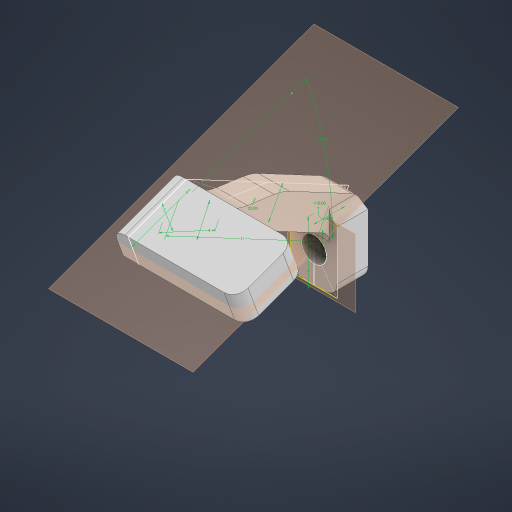
# Autodesk Inventor part: battery-stopper-1
Saved by Autodesk Inventor 2023.5 (Build 275446000, 446)
## iProperties
Created: 2025-02-09
Part Number: battery-stopper-1
Material: 一般
Document SubType Name: Modeling
Designer: IshiiLabHonda
Density: 1 g/cm^3
Appearance: 既定
Author: IshiiLabHonda
Autodesk Inventor part; units mm, degrees
ref_plane "YZ Plane" through (0, 0, 0) normal (1, 0, 0) x (0, 1, 0)
ref_plane "XZ Plane" through (0, 0, 0) normal (0, 1, 0) x (-1, 0, 0)
ref_plane "XY Plane" through (0, 0, 0) normal (0, 0, 1) x (1, 0, 0)
sketch "スケッチ5" plane through (0, 0, 0) normal (1, 0, 0) x (0, 1, 0)
  line L0 (0, 0) -> (0, 1.2936) construction
  line L1 (0, 0) -> (-1.3338, 0) construction
  line L2 (2, 2) -> (-2, 2)
  line L3 (-2, 2) -> (-2, 0)
  line L4 (-2, 0) -> (2, 0)
  line L5 (2, 0) -> (2, 2)
  line L6 (0.8, 2) -> (0.8, 0)
  line L7 (-0.8, 2) -> (-0.8, 0)
  line L8 (-2, 1) -> (2, 1) construction
  line L9 (2, 1) -> (7.1642, 10.7124) construction
  line L10 (8.0471, 10.243) -> (6.2812, 11.1819)
  line L11 (6.2812, 11.1819) -> (0.7025, 0.6899)
  line L12 (0.7025, 0.6899) -> (2.4684, -0.2491)
  line L13 (2.4684, -0.2491) -> (8.0471, 10.243)
  line L14 (2, 0) -> (2.6009, 0)
  line L15 (6.6791, 14.0017) -> (4.7997, 13.3177)
  line L16 (4.7997, 13.3177) -> (6.1677, 9.5589)
  line L17 (6.1677, 9.5589) -> (8.0471, 10.243)
  line L18 (8.0471, 10.243) -> (6.6791, 14.0017)
  line L19 (6.6791, 14.0017) -> (6.1677, 9.5589) construction
  line L20 (4.7997, 13.3177) -> (8.0471, 10.243) construction
  line L21 (5.7394, 13.6597) -> (7.1074, 9.9009) construction
  line L22 (6.4234, 11.7803) -> (4.7515, 8.1465) construction
  line L23 (4.7515, 8.1465) -> (4.3748, 5.4664) construction
  line L24 (6.2812, 11.1819) -> (2.4684, -0.2491) construction
  line L25 (0.7025, 0.6899) -> (8.0471, 10.243) construction
  line L26 (7.3319, 11.3623) -> (5.5149, 12.1983)
  line L27 (5.5149, 12.1983) -> (3.843, 8.5645)
  line L28 (3.843, 8.5645) -> (5.66, 7.7285)
  line L29 (5.66, 7.7285) -> (7.3319, 11.3623)
  line L30 (7.3319, 11.3623) -> (3.843, 8.5645) construction
  line L31 (5.5149, 12.1983) -> (5.66, 7.7285) construction
  line L32 (5.66, 7.7285) -> (5.2826, 5.0437)
  line L33 (3.843, 8.5645) -> (2.6532, 0.0985)
  line L34 (3.467, 5.8892) -> (5.2329, 4.9502)
  point P0 (1.3991, 2)
  point P1 (5.5874, 9.9634)
  point P2 (5.3431, 11.8247)
  point P3 (6.5694, 9.7051)
  dimension "d25" = 1.6
  dimension "d26" = 4
  dimension "d27" = 2
  dimension "d28" = 118
  dimension "d29" = 2
  dimension "d30" = 11
  dimension "d44" = 2
  dimension "d45" = 20
  dimension "d46" = 4
  dimension "d52" = 20
  dimension "d53" = 4
  dimension "d54" = 2
  constraints: 70 end point, 15 midpoint, 15 point on line, 10 parallel, 7 perpendicular, 1 coincident, 1 vertical, 6 other
  measures "d25" distance between parallel lines of L7 L6
  measures "d26" distance between parallel lines of L3 L5
  measures "d27" distance between parallel lines of L4 L2
  measures "d28" angle of L8 L9
  measures "d29" distance between parallel lines of L13 L11
  measures "d30" distance of L8.end L9.end
  measures "d44" distance between parallel lines of L18 L16
  measures "d45" angle of L0 L21
  measures "d46" distance between parallel lines of L17 L15
  measures "d52" angle of L9 L23
  measures "d53" distance of L22.start L22.end
  measures "d54" distance between parallel lines of L29 L27
extrude "押し出し8" add sketch "スケッチ5" along normal mid plane 3 contours L6 L11 L12 L4 L7 L2 | L2 L11 L6 | L7 L4 L3 L2 | L2 L5 L12 L6 L11 | L6 L12 L11 | L12 L4 L6
ref_plane "作業平面7" through (-1.5, -2, 2) normal (0, 0, 1) x (1, 0, 0)
sketch "スケッチ6" plane through (-1.5, -2, 2) normal (0, 0, 1) x (1, 0, 0)
  line L0 (3, 0) -> (0, 0) projected
  line L1 (3, 4) -> (3, 0) projected
  line L2 (0, 4) -> (3, 4) projected
  line L3 (0, 0) -> (0, 4) projected
  line L4 (0, 4) -> (3, 4) projected
  line L5 (0, 4) -> (3, 0) construction
  line L6 (0, 0) -> (3, 0) projected
  line L7 (3, 0) -> (3, 4) projected
  line L8 (0, 0) -> (3, 4) construction
  circle A0 centre (1.5, 2) radius 0.8
  dimension "d35" = 1.6
  constraints: 4 end point, 1 centre point, 1 coincident
  measures "d35" diameter of A0
extrude "押し出し9" cut sketch "スケッチ6" against normal blind 4 contours A0
extrude "押し出し13" add sketch "スケッチ5" along normal blind 7 contours L16 L27 L26 L29 L10 L11 | L11 L10 L29 L17 L16 | L16 L15 L18 L10 L29 L26 L27 | L29 L10 L17
extrude "押し出し15" add sketch "スケッチ5" along normal mid plane 2 contours L11 L33 L13 L14 L5 L2 | L33 L28 L11 | L34 L13 L33 | L11 L28 L32 L13 L34 | L28 L27 L16 L11 | L11 L16 L17 L29 L28 | L16 L27 L26 L29 L10 L11 | L11 L10 L29 L17 L16
extrude "押し出し16" add sketch "スケッチ5" against normal blind 1 contours L16 L15 L18 L10 L29 L26 L27 | L29 L10 L17
fillet "フィレット1" radius 0.8 1 edges at (0, 1.3991, 2)
fillet "フィレット2" radius 1 1 edges at (0, 2.6009, 0)
fillet "フィレット3" radius 3 4 edges at (0, 5.2826, 5.0437) (0, 3.467, 5.8892) (0, 3.843, 8.5645) (0, 5.66, 7.7285)
fillet "フィレット4" radius 3 2 edges at (0, 5.3431, 11.8247) (0, 6.5694, 9.7051)
fillet "フィレット6" radius 0.8 1 edges at (-1, 7.3631, 12.1223)
ref_plane "作業平面8" through (-0.2, 5.7394, 13.6597) normal (0, 0.9396926, 0.3420201) x (1, 0, 0)
sketch "スケッチ8" plane through (-0.2, 5.7394, 13.6597) normal (0, 0.9396926, 0.3420201) x (1, 0, 0)
  point P0 (0.2, 10.8729)
fillet "フィレット11" radius 0.8 2 edges at (7, 5.7394, 13.6597) (7, 7.1074, 9.9009)
fillet "フィレット12" radius 0.8 4 edges at (1, 2, 1) (-1, 2, 1) (-1.5, -2, 1) (1.5, -2, 1)
fillet "フィレット13" radius 0.4 1 edges at (1, 5.5444, 11.2714)
